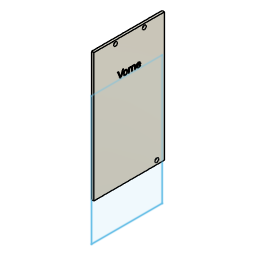
Assembly CanSat EV v2 (Autodesk Fusion 360 archive; units mm, degrees)
design "Energieversorgung"
Autodesk Fusion 360 part; units mm, degrees
sketch "Skizze1" plane through (0, 0, 0) normal (1, 0, 0) x (0, 1, 0)
  line L0 (-25, -30) -> (30, -30)
  line L1 (30, -30) -> (30, 70)
  line L2 (30, 70) -> (-25, 70)
  line L3 (-25, 70) -> (-25, -30)
  dimension "d1" = 55
  dimension "d2" = 100
  constraint horizontal L0
  constraint vertical L1
  constraint horizontal L2
  constraint vertical L3
  measures "d1" distance of L0.start L0.end
  measures "d2" distance of L0 L2
extrude "Extrusion1" add sketch "Skizze1" along normal blind 1.8
move_body "Verschieben1" bodies 1 to x (1, 0, 0) y (0, 1, 0) z (0, 0, 1) at (0, 0, 30)
sketch "Skizze2" plane through (1.8, 0, 0) normal (1, 0, 0) x (0, 1, 0)
  line L0 (-25, 100) -> (-25, 0)
  line L1 (-25, 0) -> (30, 0)
  line L2 (30, 0) -> (30, 100)
  line L3 (30, 100) -> (-25, 100)
  circle A0 centre (14.32, 97.38) radius 1.5
  circle A1 centre (-8.13, 97.4) radius 1.5
  circle A2 centre (23.99, 3.06) radius 1.5
  line L4 (-15, 65) -> (20, 65) construction
  line L5 (20, 65) -> (20, 85) construction
  line L6 (20, 85) -> (-15, 85) construction
  line L7 (-15, 85) -> (-15, 65) construction
  dimension "d5" = 3
  dimension "d6" = 3
  dimension "d7" = 3
  dimension "d14" = 2.62
  dimension "d15" = 15.68
  dimension "d16" = 16.87
  dimension "d17" = 2.6
  dimension "d18" = 6.01
  dimension "d19" = 3.06
  dimension "d22" = 5
  text T0 "Vorne" font "Arial" height 5 align centre middle in box 35 x 20 at (-15, 65) x (1, 0) y (0, 1) spacing 1 kerned
  measures "d5" diameter of A0
  measures "d6" diameter of A1
  measures "d7" diameter of A2
  measures "d14" distance of L3 A0.centre
  measures "d15" distance of L2 A0.centre
  measures "d16" distance of L0 A1.centre
  measures "d17" distance of L3 A1.centre
  measures "d18" distance of L2 A2.centre
  measures "d19" distance of L1 A2.centre
extrude "Extrusion4" cut sketch "Skizze2" against normal blind 11 contours A0 | A1 | A2
extrude "Extrusion2" cut sketch "Skizze2" against normal blind 10 contours A0 | A1 | A2
extrude "Extrusion3" cut sketch "Skizze2" against normal blind 1 text T0

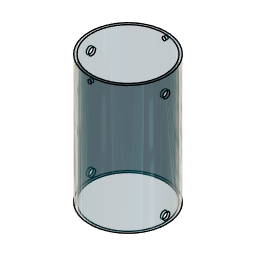
design "Mantel EV"
Autodesk Fusion 360 part; units mm, degrees
sketch "Skizze1" plane through (0, 0, 0) normal (0, 0, 1) x (1, 0, 0)
  circle A0 centre (0, 0) radius 33
  circle A1 centre (0, 0) radius 31
  dimension "d1" = 66
  dimension "d2" = 62
  constraint coincident A0.centre A1.centre
  measures "d1" diameter of A0
  measures "d2" diameter of A1
extrude "Extrusion1" add sketch "Skizze1" along normal blind 110
ref_plane "Arbeitsebene1" through (33, 0, 78.9185) normal (1, 0, 0) x (0, -1, 0)
sketch "Skizze2" plane through (33, 0, 0) normal (1, 0, 0) x (0, 1, 0)
  circle A0 centre (0, 6.05) radius 3
  circle A1 centre (0, 96.45) radius 3
  dimension "d6" = 6
  dimension "d7" = 6.05
  dimension "d8" = 6
  dimension "d9" = 90.4
  measures "d6" diameter of A0
  measures "d7" distance of origin A0.centre
  measures "d8" diameter of A1
  measures "d9" distance of A0.centre A1.centre
extrude "Extrusion2" cut sketch "Skizze2" against normal blind 85
ref_plane "Arbeitsebene2" through (0, -33, 86.9154) normal (0, -1, 0) x (-1, 0, 0)
sketch "Skizze3" plane through (0, -33, 0) normal (0, -1, 0) x (-1, 0, 0)
  circle A0 centre (0, -105.95) radius 1.5
  line L0 (33, -110) -> (-33, -110) construction
  dimension "d13" = 3
  dimension "d14" = 4.05
  constraint horizontal L0
  measures "d13" diameter of A0
  measures "d14" distance of A0.centre L0
extrude "Extrusion3" cut sketch "Skizze3" against normal blind 75
equation "d9 = 84.4 mm + 6 mm"
